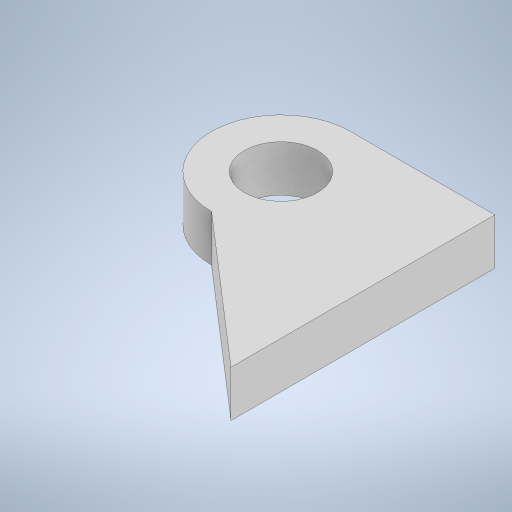
# Autodesk Inventor part: TrubaDerzanka
Saved by Autodesk Inventor 2024 (Build 280153000, 153)
## iProperties
Created: 2023-08-21
Part Number: TrubaDerzanka
Material: Generic
Document SubType Name: Modeling
Designer: KirikDK
Density: 1 g/cm^3
Appearance: Default
Author: KirikDK
Autodesk Inventor part; units mm, degrees
ref_plane "YZ Plane" through (0, 0, 0) normal (1, 0, 0) x (0, 1, 0)
ref_plane "XZ Plane" through (0, 0, 0) normal (0, 1, 0) x (-1, 0, 0)
ref_plane "XY Plane" through (0, 0, 0) normal (0, 0, 1) x (1, 0, 0)
sketch "Sketch1" plane through (0, 0, 0) normal (0, 1, 0) x (-1, 0, 0)
  circle A0 centre (31.197, 0) radius 7.9
  line L0 (46.197, 15) -> (0, 15)
  line L1 (0, 15) -> (0, -15)
  line L2 (0, -15) -> (46.197, -15)
  line L3 (46.197, -15) -> (46.197, 15)
  circle A1 centre (31.197, 0) radius 15
  line L4 (46.197, 15) -> (0, 15)
  line L5 (0, 15) -> (0, 42)
  line L6 (0, 42) -> (46.197, 42)
  line L7 (46.197, 42) -> (46.197, 15)
  line L8 (31.197, 15) -> (0, 42)
  point P0 (0, 0)
  point P1 (0, 0)
  point P2 (31.197, -15)
  dimension "d0" = 15.8
  dimension "d1" = 31.197
  dimension "d2" = 42
  constraints: 18 end point, 4 horizontal, 4 parallel, 2 perpendicular, 1 centre point, 1 coincident, 1 midpoint, 1 point on line, 1 vertical, 3 other
  measures "d0" diameter of A0
  measures "d1" distance of point (0, 0) A0.centre
  measures "d2" distance from line of L6 A0.centre
extrude "Extrusion1" add sketch "Sketch1" along normal blind 10 contours A1 L2 L1 L0 | A1 | L0 L5 L8
body "Solid1"
